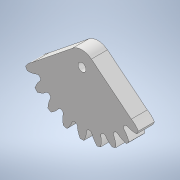
# Autodesk Inventor part: Pinion222
Saved by Autodesk Inventor 2022 (Build 260153000, 153)
## iProperties
Created: 2022-06-04
Part Number: Pinion222
Material: Generic
Document SubType Name: Modeling
Designer: frede
Density: 1 g/cm^3
Appearance: Default
Author: frede
Autodesk Inventor part; units mm, degrees
(part 1 of 2)
ref_plane "YZ Plane" through (0, 0, 0) normal (1, 0, 0) x (0, 1, 0)
ref_plane "XZ Plane" through (0, 0, 0) normal (0, 1, 0) x (-1, 0, 0)
ref_plane "XY Plane" through (0, 0, 0) normal (0, 0, 1) x (1, 0, 0)
sketch "Sketch1" plane through (0, 0, 0) normal (0, 0, 1) x (1, 0, 0)
  spline S0 degree 3 poles (-3.3489, 31.0344) (-3.2669, 30.9208) (-3.1027, 30.6937) (-2.8692, 30.344) (-2.6455, 29.988) (-2.4333, 29.625) (-2.2335, 29.255) (-2.0474, 28.8779) (-1.8767, 28.4936) (-1.7233, 28.102) (-1.5918, 27.7027) (-1.4824, 27.296) (-1.4363, 26.9482) (-1.3713, 26.6753) (-1.3031, 26.4761) (-1.2148, 26.2851) (-1.1055, 26.1048) (-0.9893, 25.973) (-0.8874, 25.8765) (-0.8022, 25.8147) (-0.714, 25.7572) (-0.6186, 25.7128) (-0.5212, 25.6728) (-0.4188, 25.6481) (-0.3154, 25.6283) (-0.1751, 25.6229) (0, 25.6264) (0.1751, 25.6229) (0.3154, 25.6283) (0.4188, 25.6481) (0.5212, 25.6728) (0.6186, 25.7128) (0.714, 25.7572) (0.8022, 25.8147) (0.8874, 25.8765) (0.9893, 25.973) (1.1055, 26.1048) (1.2148, 26.2851) (1.3031, 26.4761) (1.3713, 26.6753) (1.4363, 26.9482) (1.4824, 27.296) (1.5918, 27.7027) (1.7233, 28.102) (1.8767, 28.4936) (2.0474, 28.8779) (2.2335, 29.255) (2.4333, 29.625) (2.6455, 29.988) (2.8692, 30.344) (3.1027, 30.6937) (3.2669, 30.9208) (3.3489, 31.0344) knots 0 0 0 0 0.042039 0.084079 0.126119 0.168158 0.210197 0.252236 0.294274 0.336311 0.378346 0.420376 0.46241 0.483428 0.504444 0.525453 0.546459 0.567453 0.577965 0.588475 0.598984 0.609494 0.620001 0.63051 0.641019 0.651526 0.672547 0.693567 0.704074 0.714583 0.725092 0.735599 0.746109 0.756618 0.767128 0.77764 0.798635 0.81964 0.840649 0.861665 0.882683 0.924717 0.966747 1.008782 1.050819 1.092857 1.134896 1.176935 1.218975 1.261014 1.303054 1.345093 1.345093 1.345093 1.345093
  circle A0 centre (0, 0) radius 25.625 construction
  circle A1 centre (0, 0) radius 27.0162 construction
  circle A2 centre (0, 0) radius 28.75 construction
  circle A3 centre (0, 0) radius 31.2146
  point P0 (-3.1048, 30.6922)
  point P1 (-2.8708, 30.3429)
  point P2 (-2.6474, 29.9868)
  point P3 (-2.4354, 29.6238)
  point P4 (-2.2358, 29.2538)
  point P5 (-2.05, 28.8767)
  point P6 (-1.8796, 28.4924)
  point P7 (-1.7269, 28.1007)
  point P8 (-1.5955, 27.7015)
  point P9 (-1.4914, 27.2943)
  point P10 (-1.4177, 26.8804)
  point P11 (-1.368, 26.6762)
  point P12 (-1.2997, 26.4774)
  point P13 (-1.2113, 26.2869)
  point P14 (-1.1005, 26.1085)
  point P15 (-0.9631, 25.9497)
  point P16 (-0.8859, 25.8783)
  point P17 (-0.8017, 25.8154)
  point P18 (-0.7128, 25.7594)
  point P19 (-0.6182, 25.7135)
  point P20 (-0.5203, 25.6754)
  point P21 (-0.4186, 25.6489)
  point P22 (-0.3151, 25.6309)
  point P23 (-0.2102, 25.6249)
  point P24 (0, 25.625)
  point P25 (0.2102, 25.6249)
  point P26 (0.3151, 25.6309)
  point P27 (0.4186, 25.6489)
  point P28 (0.5203, 25.6754)
  point P29 (0.6182, 25.7135)
  point P30 (0.7128, 25.7594)
  point P31 (0.8017, 25.8154)
  point P32 (0.8859, 25.8783)
  point P33 (0.9631, 25.9497)
  point P34 (1.1005, 26.1085)
  point P35 (1.2113, 26.2869)
  point P36 (1.2997, 26.4774)
  point P37 (1.368, 26.6762)
  point P38 (1.4177, 26.8804)
  point P39 (1.4914, 27.2943)
  point P40 (1.5955, 27.7015)
  point P41 (1.7269, 28.1007)
  point P42 (1.8796, 28.4924)
  point P43 (2.05, 28.8767)
  point P44 (2.2358, 29.2538)
  point P45 (2.4354, 29.6238)
  point P46 (2.6474, 29.9868)
  point P47 (2.8708, 30.3429)
  point P48 (3.1048, 30.6922)
  constraints: 4 centre point, 2 point on circle, 107 other
extrude "Extrusion1" add sketch "Sketch1" against normal blind 8
extrude "Extrusion2" cut sketch "Sketch1" against normal through all contours A3 S0 picked at (-0.4102, 29.7407)
pattern_circular "Circular Pattern1" count 23 over 360 about axis through (0, 0, 0) along (0, 0, -1) of "Extrusion2"
sketch "Sketch3" plane through (0, 0, 0) normal (0, 0, 1) x (1, 0, 0)
  circle A0 centre (0, 0) radius 2
  dimension "d16" = 4
  constraints: 1 centre point, 1 coincident
  measures "d16" diameter of A0
extrude "Extrusion4" cut sketch "Sketch3" against normal through all
sketch "Sketch4" plane through (0, 0, -8) normal (0, 0, -1) x (-1, 0, 0)
  circle A0 centre (0, 0) radius 2 projected
  arc A1 (7.5436, -30.2893) -> (9.2925, -29.7993) centre (0, 0) ccw projected
  line L0 (0, 0) -> (0.9081, -31.2014) construction
  line L1 (0, 0) -> (26.1697, 16.142) construction
  circle A2 centre (0, 0) radius 7.5 construction
  circle A3 centre (0, 0) radius 2 projected
  spline S0 degree 5 poles (11.5977, 28.98) (11.5528, 28.9443) (11.5079, 28.9087) (11.4631, 28.8729) (11.3736, 28.8011) (11.2848, 28.7285) (11.2406, 28.692) (11.1527, 28.6184) (11.0656, 28.5437) (11.0223, 28.5061) (10.936, 28.4305) (10.8504, 28.3541) (10.8079, 28.3157) (10.7231, 28.2384) (10.6391, 28.1603) (10.5973, 28.121) (10.5142, 28.0419) (10.432, 27.962) (10.3911, 27.9218) (10.3097, 27.8409) (10.2294, 27.759) (10.1894, 27.7179) (10.1101, 27.6351) (10.0317, 27.5513) (9.9928, 27.5092) (9.9155, 27.4244) (9.8393, 27.3386) (9.8015, 27.2955) (9.7265, 27.2087) (9.6527, 27.1209) (9.6161, 27.0768) (9.5435, 26.9879) (9.4724, 26.898) (9.4371, 26.8527) (9.3674, 26.7616) (9.2993, 26.6693) (9.2655, 26.623) (9.1992, 26.5294) (9.1345, 26.4347) (9.1026, 26.387) (9.0395, 26.2912) (8.9784, 26.1941) (8.9484, 26.1452) (8.8896, 26.0467) (8.8341, 25.9463) (8.8071, 25.8957) (8.7566, 25.7927) (8.7081, 25.6886) (8.684, 25.6366) (8.6345, 25.533) (8.5814, 25.4313) (8.5535, 25.3811) (8.4945, 25.2826) (8.4291, 25.1882) (8.3946, 25.1423) (8.3227, 25.0526) (8.2443, 24.9687) (8.2037, 24.9279) (8.1183, 24.8511) (8.0248, 24.7838) (7.9755, 24.7547) (7.8775, 24.6942) (7.7704, 24.6518) (7.7164, 24.6331) (7.606, 24.5997) (7.4918, 24.5879) (7.4348, 24.5781) (7.32, 24.5847) (7.2058, 24.5928) (7.1497, 24.6085) (7.0395, 24.6378) (6.9295, 24.6711) (6.8743, 24.6853) (6.7637, 24.716) (6.6539, 24.7472) (6.5994, 24.7666) (6.4983, 24.8195) (6.3987, 24.8764) (6.3567, 24.9157) (6.2653, 24.9849) (6.1928, 25.0743) (6.1549, 25.1166) (6.0903, 25.2116) (6.0377, 25.3129) (6.0124, 25.3644) (5.9686, 25.4703) (5.9381, 25.5807) (5.9249, 25.6363) (5.9027, 25.7487) (5.8891, 25.8623) (5.8842, 25.9193) (5.8782, 26.0336) (5.8798, 26.1481) (5.8824, 26.2052) (5.8906, 26.3193) (5.9025, 26.4331) (5.909, 26.4899) (5.9215, 26.6036) (5.931, 26.7175) (5.934, 26.7746) (5.9383, 26.8889) (5.939, 27.0032) (5.9386, 27.0604) (5.9366, 27.1747) (5.9323, 27.2889) (5.9297, 27.346) (5.9234, 27.4601) (5.9152, 27.5741) (5.9104, 27.631) (5.9, 27.7448) (5.8876, 27.8584) (5.881, 27.9151) (5.8669, 28.0285) (5.851, 28.1417) (5.8426, 28.1982) (5.8251, 28.3111) (5.8061, 28.4238) (5.7962, 28.4801) (5.7756, 28.5925) (5.7537, 28.7046) (5.7423, 28.7606) (5.7189, 28.8725) (5.6941, 28.984) (5.6814, 29.0397) (5.6553, 29.1509) (5.6279, 29.2619) (5.6139, 29.3173) (5.5852, 29.4279) (5.5553, 29.5382) (5.5401, 29.5932) (5.509, 29.7032) (5.4768, 29.8128) (5.4604, 29.8676) (5.4271, 29.9769) (5.3928, 30.0859) (5.3754, 30.1403) (5.3399, 30.2489) (5.3031, 30.3571) (5.2844, 30.4111) (5.2464, 30.5188) (5.2074, 30.6262) (5.1877, 30.6799) (5.168, 30.7335) (5.1482, 30.7871) knots 0 0 0 0 0 0 0.021315 0.021315 0.021315 0.04263 0.04263 0.04263 0.063945 0.063945 0.063945 0.08526 0.08526 0.08526 0.106575 0.106575 0.106575 0.12789 0.12789 0.12789 0.149204 0.149204 0.149204 0.170519 0.170519 0.170519 0.191835 0.191835 0.191835 0.21315 0.21315 0.21315 0.234465 0.234465 0.234465 0.255779 0.255779 0.255779 0.277094 0.277094 0.277094 0.298412 0.298412 0.298412 0.319724 0.319724 0.319724 0.341052 0.341052 0.341052 0.362374 0.362374 0.362374 0.383705 0.383705 0.383705 0.405045 0.405045 0.405045 0.42637 0.42637 0.42637 0.447676 0.447676 0.447676 0.468973 0.468973 0.468973 0.490261 0.490261 0.490261 0.511544 0.511544 0.511544 0.532795 0.532795 0.532795 0.554 0.554 0.554 0.575212 0.575212 0.575212 0.596458 0.596458 0.596458 0.617711 0.617711 0.617711 0.63897 0.63897 0.63897 0.660221 0.660221 0.660221 0.681474 0.681474 0.681474 0.702716 0.702716 0.702716 0.723962 0.723962 0.723962 0.745198 0.745198 0.745198 0.76643 0.76643 0.76643 0.787663 0.787663 0.787663 0.808897 0.808897 0.808897 0.830131 0.830131 0.830131 0.851365 0.851365 0.851365 0.872598 0.872598 0.872598 0.893831 0.893831 0.893831 0.915065 0.915065 0.915065 0.936299 0.936299 0.936299 0.957533 0.957533 0.957533 0.978766 0.978766 0.978766 1 1 1 1 1 1 projected
  arc A4 (5.1482, 30.7871) -> (3.3489, 31.0344) centre (0, 0) ccw projected
  spline S1 degree 5 poles (3.3489, 31.0344) (3.3153, 30.9879) (3.2817, 30.9415) (3.2482, 30.8949) (3.1814, 30.8017) (3.1155, 30.7078) (3.0828, 30.6607) (3.018, 30.5661) (2.9543, 30.4707) (2.9227, 30.4228) (2.86, 30.3267) (2.7982, 30.2301) (2.7676, 30.1816) (2.7068, 30.0843) (2.647, 29.9864) (2.6174, 29.9373) (2.5587, 29.8388) (2.5011, 29.7396) (2.4725, 29.6898) (2.416, 29.59) (2.3607, 29.4895) (2.3334, 29.4391) (2.2793, 29.3379) (2.2265, 29.2361) (2.2004, 29.1851) (2.1488, 29.0826) (2.0986, 28.9795) (2.0738, 28.9277) (2.025, 28.8239) (1.9776, 28.7195) (1.9543, 28.6671) (1.9084, 28.5619) (1.8641, 28.4561) (1.8424, 28.403) (1.7998, 28.2965) (1.7591, 28.1893) (1.7392, 28.1355) (1.7005, 28.0275) (1.6638, 27.9189) (1.6459, 27.8644) (1.611, 27.7551) (1.5784, 27.6451) (1.5627, 27.5899) (1.5327, 27.4792) (1.5063, 27.3676) (1.494, 27.3115) (1.4731, 27.1987) (1.4545, 27.0855) (1.4453, 27.0288) (1.4256, 26.9158) (1.4019, 26.8035) (1.3885, 26.7476) (1.3583, 26.6369) (1.3208, 26.5283) (1.2999, 26.4748) (1.2549, 26.369) (1.2021, 26.2671) (1.174, 26.2168) (1.1125, 26.1199) (1.0407, 26.0298) (1.001, 25.9885) (0.923, 25.9038) (0.8313, 25.8341) (0.7843, 25.8015) (0.6871, 25.7395) (0.5802, 25.6974) (0.528, 25.6726) (0.4156, 25.648) (0.3035, 25.625) (0.2453, 25.6249) (0.1313, 25.6234) (0.0163, 25.6258) (-0.0407, 25.6246) (-0.1554, 25.6243) (-0.2695, 25.6247) (-0.3273, 25.6287) (-0.4389, 25.6524) (-0.5501, 25.6803) (-0.6012, 25.7068) (-0.7079, 25.7487) (-0.8018, 25.8153) (-0.8498, 25.8458) (-0.9376, 25.9198) (-1.0156, 26.0032) (-1.0538, 26.046) (-1.1245, 26.1361) (-1.1837, 26.2342) (-1.2114, 26.2842) (-1.2631, 26.3864) (-1.3068, 26.4921) (-1.3269, 26.5457) (-1.3636, 26.6542) (-1.3929, 26.7648) (-1.4058, 26.8205) (-1.4288, 26.9326) (-1.4479, 27.0453) (-1.4571, 27.1018) (-1.4757, 27.2146) (-1.4972, 27.3269) (-1.5097, 27.3827) (-1.5364, 27.4939) (-1.5667, 27.6042) (-1.5824, 27.6591) (-1.6152, 27.7686) (-1.6502, 27.8775) (-1.6681, 27.9317) (-1.7049, 28.0399) (-1.7435, 28.1474) (-1.7635, 28.201) (-1.8042, 28.3077) (-1.8468, 28.4138) (-1.8685, 28.4666) (-1.9127, 28.572) (-1.9585, 28.6767) (-1.9818, 28.7289) (-2.0291, 28.8329) (-2.0779, 28.9362) (-2.1026, 28.9877) (-2.1527, 29.0904) (-2.2041, 29.1925) (-2.2302, 29.2433) (-2.2829, 29.3447) (-2.3368, 29.4455) (-2.3641, 29.4956) (-2.4193, 29.5957) (-2.4756, 29.6951) (-2.504, 29.7447) (-2.5615, 29.8435) (-2.62, 29.9416) (-2.6495, 29.9905) (-2.7091, 30.088) (-2.7697, 30.1849) (-2.8002, 30.2332) (-2.8618, 30.3295) (-2.9243, 30.4252) (-2.9557, 30.4729) (-3.0192, 30.5679) (-3.0838, 30.6621) (-3.1164, 30.7091) (-3.1821, 30.8026) (-3.2486, 30.8955) (-3.282, 30.9418) (-3.3155, 30.9881) (-3.3489, 31.0344) knots 0 0 0 0 0 0 0.021315 0.021315 0.021315 0.04263 0.04263 0.04263 0.063945 0.063945 0.063945 0.08526 0.08526 0.08526 0.106575 0.106575 0.106575 0.12789 0.12789 0.12789 0.149204 0.149204 0.149204 0.170519 0.170519 0.170519 0.191835 0.191835 0.191835 0.21315 0.21315 0.21315 0.234465 0.234465 0.234465 0.255779 0.255779 0.255779 0.277094 0.277094 0.277094 0.298412 0.298412 0.298412 0.319724 0.319724 0.319724 0.341052 0.341052 0.341052 0.362374 0.362374 0.362374 0.383705 0.383705 0.383705 0.405045 0.405045 0.405045 0.42637 0.42637 0.42637 0.447676 0.447676 0.447676 0.468973 0.468973 0.468973 0.490261 0.490261 0.490261 0.511544 0.511544 0.511544 0.532795 0.532795 0.532795 0.554 0.554 0.554 0.575212 0.575212 0.575212 0.596458 0.596458 0.596458 0.617711 0.617711 0.617711 0.63897 0.63897 0.63897 0.660221 0.660221 0.660221 0.681474 0.681474 0.681474 0.702716 0.702716 0.702716 0.723962 0.723962 0.723962 0.745198 0.745198 0.745198 0.76643 0.76643 0.76643 0.787663 0.787663 0.787663 0.808897 0.808897 0.808897 0.830131 0.830131 0.830131 0.851365 0.851365 0.851365 0.872598 0.872598 0.872598 0.893831 0.893831 0.893831 0.915065 0.915065 0.915065 0.936299 0.936299 0.936299 0.957533 0.957533 0.957533 0.978766 0.978766 0.978766 1 1 1 1 1 1 projected
  arc A5 (-3.3489, 31.0344) -> (-5.1482, 30.7871) centre (0, 0) ccw projected
  spline S2 degree 5 poles (-5.1482, 30.7871) (-5.168, 30.7333) (-5.1879, 30.6795) (-5.2076, 30.6256) (-5.2468, 30.5178) (-5.2849, 30.4096) (-5.3037, 30.3554) (-5.3406, 30.2468) (-5.3762, 30.1378) (-5.3936, 30.0832) (-5.4281, 29.9737) (-5.4615, 29.864) (-5.4779, 29.8091) (-5.5102, 29.699) (-5.5414, 29.5886) (-5.5567, 29.5333) (-5.5866, 29.4226) (-5.6153, 29.3115) (-5.6294, 29.2559) (-5.6568, 29.1446) (-5.683, 29.0329) (-5.6957, 28.977) (-5.7205, 28.865) (-5.7439, 28.7527) (-5.7553, 28.6965) (-5.7773, 28.5839) (-5.7978, 28.471) (-5.8077, 28.4145) (-5.8267, 28.3014) (-5.8442, 28.188) (-5.8525, 28.1313) (-5.8683, 28.0177) (-5.8824, 27.9038) (-5.889, 27.8468) (-5.9012, 27.7328) (-5.9115, 27.6186) (-5.9162, 27.5614) (-5.9243, 27.447) (-5.9304, 27.3324) (-5.9329, 27.2751) (-5.9369, 27.1605) (-5.9387, 27.0458) (-5.9389, 26.9884) (-5.938, 26.8737) (-5.9332, 26.7591) (-5.93, 26.7018) (-5.9197, 26.5875) (-5.907, 26.4735) (-5.9006, 26.4165) (-5.889, 26.3023) (-5.8816, 26.1877) (-5.8794, 26.1304) (-5.8786, 26.0156) (-5.8854, 25.9009) (-5.8911, 25.8438) (-5.9059, 25.7298) (-5.9293, 25.6174) (-5.9428, 25.5614) (-5.9758, 25.4514) (-6.0207, 25.3453) (-6.0477, 25.2948) (-6.1, 25.1922) (-6.1695, 25.1004) (-6.2059, 25.0563) (-6.2829, 24.9704) (-6.3743, 24.901) (-6.418, 24.863) (-6.5195, 24.809) (-6.6213, 24.7566) (-6.6773, 24.7409) (-6.7867, 24.7086) (-6.898, 24.6799) (-6.9526, 24.6634) (-7.063, 24.6321) (-7.173, 24.6018) (-7.2297, 24.59) (-7.3435, 24.5827) (-7.4582, 24.5796) (-7.5146, 24.5913) (-7.6285, 24.6029) (-7.7369, 24.6416) (-7.7914, 24.6581) (-7.8959, 24.7057) (-7.9935, 24.7649) (-8.0418, 24.7958) (-8.1342, 24.8635) (-8.2177, 24.942) (-8.2579, 24.9827) (-8.3352, 25.0671) (-8.4059, 25.1571) (-8.4397, 25.2033) (-8.5042, 25.2979) (-8.5623, 25.3965) (-8.5898, 25.4467) (-8.6421, 25.5484) (-8.691, 25.6518) (-8.715, 25.7037) (-8.7634, 25.8073) (-8.8144, 25.9096) (-8.8415, 25.96) (-8.8972, 26.0598) (-8.9561, 26.1579) (-8.9861, 26.2065) (-9.0472, 26.3031) (-9.1102, 26.3985) (-9.1421, 26.4459) (-9.2067, 26.5401) (-9.273, 26.6333) (-9.3066, 26.6794) (-9.3747, 26.7712) (-9.4443, 26.8619) (-9.4794, 26.9069) (-9.5504, 26.9964) (-9.6228, 27.0849) (-9.6593, 27.1288) (-9.7329, 27.2162) (-9.8077, 27.3026) (-9.8454, 27.3455) (-9.9214, 27.4309) (-9.9984, 27.5153) (-10.0372, 27.5572) (-10.1153, 27.6406) (-10.1944, 27.7231) (-10.2343, 27.764) (-10.3144, 27.8455) (-10.3954, 27.9261) (-10.4362, 27.9661) (-10.5182, 28.0457) (-10.601, 28.1244) (-10.6426, 28.1636) (-10.7263, 28.2414) (-10.8108, 28.3183) (-10.8532, 28.3566) (-10.9385, 28.4327) (-11.0244, 28.5079) (-11.0676, 28.5454) (-11.1543, 28.6198) (-11.242, 28.6931) (-11.286, 28.7295) (-11.3745, 28.8018) (-11.4636, 28.8733) (-11.5083, 28.9089) (-11.553, 28.9445) (-11.5977, 28.98) knots 0 0 0 0 0 0 0.021315 0.021315 0.021315 0.04263 0.04263 0.04263 0.063945 0.063945 0.063945 0.08526 0.08526 0.08526 0.106575 0.106575 0.106575 0.12789 0.12789 0.12789 0.149204 0.149204 0.149204 0.170519 0.170519 0.170519 0.191835 0.191835 0.191835 0.21315 0.21315 0.21315 0.234465 0.234465 0.234465 0.255779 0.255779 0.255779 0.277094 0.277094 0.277094 0.298412 0.298412 0.298412 0.319724 0.319724 0.319724 0.341052 0.341052 0.341052 0.362374 0.362374 0.362374 0.383705 0.383705 0.383705 0.405045 0.405045 0.405045 0.42637 0.42637 0.42637 0.447676 0.447676 0.447676 0.468973 0.468973 0.468973 0.490261 0.490261 0.490261 0.511544 0.511544 0.511544 0.532795 0.532795 0.532795 0.554 0.554 0.554 0.575212 0.575212 0.575212 0.596458 0.596458 0.596458 0.617711 0.617711 0.617711 0.63897 0.63897 0.63897 0.660221 0.660221 0.660221 0.681474 0.681474 0.681474 0.702716 0.702716 0.702716 0.723962 0.723962 0.723962 0.745198 0.745198 0.745198 0.76643 0.76643 0.76643 0.787663 0.787663 0.787663 0.808897 0.808897 0.808897 0.830131 0.830131 0.830131 0.851365 0.851365 0.851365 0.872598 0.872598 0.872598 0.893831 0.893831 0.893831 0.915065 0.915065 0.915065 0.936299 0.936299 0.936299 0.957533 0.957533 0.957533 0.978766 0.978766 0.978766 1 1 1 1 1 1 projected
  arc A6 (-11.5977, 28.98) -> (-13.2636, 28.2565) centre (0, 0) ccw projected
  spline S3 degree 5 poles (-13.2636, 28.2565) (-13.2681, 28.1993) (-13.2727, 28.1421) (-13.2772, 28.0849) (-13.2858, 27.9706) (-13.2933, 27.8561) (-13.2968, 27.7989) (-13.303, 27.6843) (-13.3079, 27.5697) (-13.31, 27.5124) (-13.3136, 27.3978) (-13.3162, 27.2831) (-13.3172, 27.2257) (-13.3186, 27.111) (-13.3188, 26.9963) (-13.3186, 26.939) (-13.3176, 26.8243) (-13.3153, 26.7096) (-13.3138, 26.6523) (-13.3102, 26.5376) (-13.3052, 26.423) (-13.3024, 26.3657) (-13.296, 26.2512) (-13.2883, 26.1368) (-13.2841, 26.0796) (-13.2749, 25.9652) (-13.2642, 25.851) (-13.2585, 25.7939) (-13.2463, 25.6799) (-13.2325, 25.566) (-13.2252, 25.5091) (-13.2098, 25.3954) (-13.1926, 25.282) (-13.1836, 25.2254) (-13.1646, 25.1123) (-13.1437, 24.9995) (-13.1328, 24.9432) (-13.1097, 24.8308) (-13.0846, 24.7189) (-13.0716, 24.663) (-13.0446, 24.5515) (-13.0153, 24.4406) (-13.0001, 24.3853) (-12.9682, 24.2751) (-12.9327, 24.166) (-12.9141, 24.1117) (-12.8734, 24.0045) (-12.8304, 23.8981) (-12.8089, 23.8449) (-12.7669, 23.7381) (-12.7289, 23.6298) (-12.7112, 23.5751) (-12.6795, 23.4648) (-12.6551, 23.3526) (-12.6452, 23.296) (-12.6287, 23.1822) (-12.6209, 23.0677) (-12.6188, 23.0101) (-12.6209, 22.8953) (-12.6355, 22.7811) (-12.6479, 22.7251) (-12.6706, 22.6123) (-12.7127, 22.5051) (-12.7359, 22.4528) (-12.7868, 22.3493) (-12.8562, 22.2578) (-12.8879, 22.2095) (-12.9711, 22.1301) (-13.055, 22.0522) (-13.1047, 22.0219) (-13.2014, 21.9613) (-13.3008, 21.9036) (-13.3489, 21.873) (-13.4467, 21.8132) (-13.5445, 21.7542) (-13.5959, 21.7276) (-13.7035, 21.6899) (-13.8131, 21.6559) (-13.8706, 21.652) (-13.9834, 21.6324) (-14.0982, 21.6405) (-14.1551, 21.6416) (-14.2686, 21.6592) (-14.3786, 21.69) (-14.4334, 21.7066) (-14.5407, 21.7469) (-14.6422, 21.7999) (-14.6919, 21.8283) (-14.7891, 21.8887) (-14.8815, 21.9564) (-14.9265, 21.9917) (-15.0141, 22.0653) (-15.0967, 22.1446) (-15.1367, 22.1855) (-15.2145, 22.2694) (-15.2895, 22.3557) (-15.3266, 22.3992) (-15.4011, 22.486) (-15.4779, 22.5707) (-15.5176, 22.6119) (-15.5981, 22.693) (-15.6813, 22.7715) (-15.7233, 22.8103) (-15.8082, 22.8868) (-15.8946, 22.9617) (-15.9381, 22.9987) (-16.0258, 23.072) (-16.1147, 23.1438) (-16.1595, 23.1792) (-16.2498, 23.2492) (-16.3413, 23.3177) (-16.3873, 23.3516) (-16.4798, 23.4187) (-16.5733, 23.4843) (-16.6203, 23.5168) (-16.7148, 23.5811) (-16.8102, 23.6441) (-16.8581, 23.6752) (-16.9542, 23.7369) (-17.0512, 23.7974) (-17.0999, 23.8273) (-17.1976, 23.8866) (-17.296, 23.9446) (-17.3454, 23.9733) (-17.4445, 24.0302) (-17.5443, 24.0858) (-17.5943, 24.1134) (-17.6948, 24.1679) (-17.7958, 24.2214) (-17.8464, 24.2478) (-17.948, 24.3002) (-18.0501, 24.3515) (-18.1013, 24.3769) (-18.2039, 24.4271) (-18.307, 24.4764) (-18.3586, 24.5009) (-18.4622, 24.5491) (-18.5664, 24.596) (-18.6186, 24.6192) (-18.7233, 24.665) (-18.8284, 24.7098) (-18.8811, 24.732) (-18.9337, 24.7542) (-18.9864, 24.7764) knots 0 0 0 0 0 0 0.021315 0.021315 0.021315 0.04263 0.04263 0.04263 0.063945 0.063945 0.063945 0.08526 0.08526 0.08526 0.106575 0.106575 0.106575 0.12789 0.12789 0.12789 0.149204 0.149204 0.149204 0.170519 0.170519 0.170519 0.191835 0.191835 0.191835 0.21315 0.21315 0.21315 0.234465 0.234465 0.234465 0.255779 0.255779 0.255779 0.277094 0.277094 0.277094 0.298412 0.298412 0.298412 0.319724 0.319724 0.319724 0.341052 0.341052 0.341052 0.362374 0.362374 0.362374 0.383705 0.383705 0.383705 0.405045 0.405045 0.405045 0.42637 0.42637 0.42637 0.447676 0.447676 0.447676 0.468973 0.468973 0.468973 0.490261 0.490261 0.490261 0.511544 0.511544 0.511544 0.532795 0.532795 0.532795 0.554 0.554 0.554 0.575212 0.575212 0.575212 0.596458 0.596458 0.596458 0.617711 0.617711 0.617711 0.63897 0.63897 0.63897 0.660221 0.660221 0.660221 0.681474 0.681474 0.681474 0.702716 0.702716 0.702716 0.723962 0.723962 0.723962 0.745198 0.745198 0.745198 0.76643 0.76643 0.76643 0.787663 0.787663 0.787663 0.808897 0.808897 0.808897 0.830131 0.830131 0.830131 0.851365 0.851365 0.851365 0.872598 0.872598 0.872598 0.893831 0.893831 0.893831 0.915065 0.915065 0.915065 0.936299 0.936299 0.936299 0.957533 0.957533 0.957533 0.978766 0.978766 0.978766 1 1 1 1 1 1 projected
  arc A7 (-18.9864, 24.7764) -> (-20.3952, 23.6302) centre (0, 0) ccw projected
  spline S4 degree 5 poles (-20.3952, 23.6302) (-20.3842, 23.5739) (-20.3732, 23.5176) (-20.3621, 23.4613) (-20.3395, 23.3489) (-20.3159, 23.2366) (-20.3038, 23.1806) (-20.2789, 23.0686) (-20.2526, 22.9569) (-20.2392, 22.9012) (-20.2117, 22.7898) (-20.1833, 22.6787) (-20.1688, 22.6232) (-20.1392, 22.5124) (-20.1084, 22.4019) (-20.0927, 22.3467) (-20.0608, 22.2365) (-20.0277, 22.1267) (-20.0108, 22.0719) (-19.9764, 21.9625) (-19.9407, 21.8535) (-19.9225, 21.7991) (-19.8855, 21.6905) (-19.8471, 21.5824) (-19.8276, 21.5285) (-19.7879, 21.4208) (-19.7468, 21.3138) (-19.7259, 21.2603) (-19.6834, 21.1538) (-19.6394, 21.0479) (-19.6171, 20.995) (-19.5715, 20.8898) (-19.5244, 20.7852) (-19.5004, 20.7331) (-19.4516, 20.6293) (-19.4011, 20.5263) (-19.3754, 20.475) (-19.3229, 20.373) (-19.2685, 20.272) (-19.2409, 20.2218) (-19.1848, 20.1217) (-19.1267, 20.0228) (-19.0971, 19.9736) (-19.0367, 19.8761) (-18.9731, 19.7807) (-18.9405, 19.7334) (-18.8723, 19.6411) (-18.8023, 19.5503) (-18.7672, 19.5049) (-18.6979, 19.4133) (-18.6321, 19.3193) (-18.6004, 19.2715) (-18.54, 19.1738) (-18.4863, 19.0723) (-18.4615, 19.0205) (-18.4149, 18.9154) (-18.3765, 18.8072) (-18.3589, 18.7524) (-18.33, 18.6412) (-18.3132, 18.5273) (-18.3101, 18.4701) (-18.3014, 18.3553) (-18.3131, 18.2407) (-18.3213, 18.1841) (-18.3424, 18.0707) (-18.3845, 17.9639) (-18.4021, 17.9087) (-18.4608, 17.8099) (-18.5205, 17.7122) (-18.5602, 17.6697) (-18.6369, 17.5853) (-18.7171, 17.5029) (-18.7551, 17.4604) (-18.8332, 17.3764) (-18.9114, 17.2932) (-18.9538, 17.2538) (-19.0472, 17.1884) (-19.1436, 17.1261) (-19.1978, 17.1068) (-19.3012, 17.0575) (-19.414, 17.0343) (-19.4691, 17.0201) (-19.5831, 17.0064) (-19.6973, 17.0063) (-19.7546, 17.0076) (-19.8687, 17.0174) (-19.9808, 17.0411) (-20.0363, 17.055) (-20.1462, 17.087) (-20.2534, 17.1272) (-20.3063, 17.1491) (-20.4105, 17.1963) (-20.5114, 17.2504) (-20.5609, 17.279) (-20.6585, 17.3387) (-20.754, 17.4017) (-20.8015, 17.4335) (-20.8966, 17.497) (-20.9934, 17.5579) (-21.0428, 17.5868) (-21.1422, 17.6432) (-21.2434, 17.6963) (-21.2944, 17.7223) (-21.3968, 17.7731) (-21.5002, 17.8219) (-21.5521, 17.8458) (-21.6562, 17.8927) (-21.7612, 17.9379) (-21.814, 17.9598) (-21.9198, 18.0029) (-22.0263, 18.0442) (-22.0798, 18.0644) (-22.187, 18.104) (-22.2947, 18.142) (-22.3488, 18.1606) (-22.4571, 18.197) (-22.5659, 18.2319) (-22.6204, 18.249) (-22.7297, 18.2825) (-22.8393, 18.3146) (-22.8943, 18.3303) (-23.0044, 18.3609) (-23.1148, 18.3903) (-23.1701, 18.4046) (-23.2809, 18.4326) (-23.392, 18.4593) (-23.4476, 18.4723) (-23.559, 18.4977) (-23.6707, 18.522) (-23.7266, 18.5338) (-23.8385, 18.5568) (-23.9507, 18.5786) (-24.0068, 18.5893) (-24.1192, 18.61) (-24.2318, 18.6296) (-24.2881, 18.6392) (-24.4009, 18.6577) (-24.5138, 18.6748) (-24.5704, 18.683) (-24.6835, 18.6988) (-24.7968, 18.7136) (-24.8535, 18.7208) (-24.9102, 18.728) (-24.9669, 18.7351) knots 0 0 0 0 0 0 0.021315 0.021315 0.021315 0.04263 0.04263 0.04263 0.063945 0.063945 0.063945 0.08526 0.08526 0.08526 0.106575 0.106575 0.106575 0.12789 0.12789 0.12789 0.149204 0.149204 0.149204 0.170519 0.170519 0.170519 0.191835 0.191835 0.191835 0.21315 0.21315 0.21315 0.234465 0.234465 0.234465 0.255779 0.255779 0.255779 0.277094 0.277094 0.277094 0.298412 0.298412 0.298412 0.319724 0.319724 0.319724 0.341052 0.341052 0.341052 0.362374 0.362374 0.362374 0.383705 0.383705 0.383705 0.405045 0.405045 0.405045 0.42637 0.42637 0.42637 0.447676 0.447676 0.447676 0.468973 0.468973 0.468973 0.490261 0.490261 0.490261 0.511544 0.511544 0.511544 0.532795 0.532795 0.532795 0.554 0.554 0.554 0.575212 0.575212 0.575212 0.596458 0.596458 0.596458 0.617711 0.617711 0.617711 0.63897 0.63897 0.63897 0.660221 0.660221 0.660221 0.681474 0.681474 0.681474 0.702716 0.702716 0.702716 0.723962 0.723962 0.723962 0.745198 0.745198 0.745198 0.76643 0.76643 0.76643 0.787663 0.787663 0.787663 0.808897 0.808897 0.808897 0.830131 0.830131 0.830131 0.851365 0.851365 0.851365 0.872598 0.872598 0.872598 0.893831 0.893831 0.893831 0.915065 0.915065 0.915065 0.936299 0.936299 0.936299 0.957533 0.957533 0.957533 0.978766 0.978766 0.978766 1 1 1 1 1 1 projected
  arc A8 (-24.9669, 18.7351) -> (-26.0143, 17.2513) centre (0, 0) ccw projected
  spline S5 degree 5 poles (-26.0143, 17.2513) (-25.9885, 17.2001) (-25.9627, 17.1489) (-25.9368, 17.0977) (-25.8847, 16.9955) (-25.8317, 16.8938) (-25.8049, 16.8431) (-25.7507, 16.742) (-25.6953, 16.6415) (-25.6673, 16.5915) (-25.6108, 16.4916) (-25.5535, 16.3923) (-25.5245, 16.3428) (-25.4661, 16.2441) (-25.4067, 16.146) (-25.3767, 16.0971) (-25.3162, 15.9996) (-25.2547, 15.9028) (-25.2236, 15.8546) (-25.161, 15.7585) (-25.0972, 15.6632) (-25.065, 15.6157) (-25.0001, 15.5211) (-24.934, 15.4274) (-24.9007, 15.3807) (-24.8334, 15.2878) (-24.765, 15.1957) (-24.7304, 15.15) (-24.6607, 15.0588) (-24.5898, 14.9687) (-24.554, 14.9239) (-24.4817, 14.8348) (-24.4082, 14.7468) (-24.371, 14.7031) (-24.296, 14.6163) (-24.2195, 14.5308) (-24.181, 14.4883) (-24.1029, 14.4043) (-24.0233, 14.3217) (-23.9832, 14.2808) (-23.9021, 14.1996) (-23.8195, 14.12) (-23.7778, 14.0806) (-23.6932, 14.003) (-23.6063, 13.9283) (-23.5622, 13.8916) (-23.4716, 13.8211) (-23.3796, 13.7525) (-23.3336, 13.7183) (-23.2422, 13.6488) (-23.1535, 13.576) (-23.11, 13.5385) (-23.0255, 13.4607) (-22.9464, 13.3775) (-22.9085, 13.3343) (-22.8353, 13.2457) (-22.7691, 13.1519) (-22.7374, 13.1038) (-22.6796, 13.0046) (-22.6327, 12.8994) (-22.6142, 12.8451) (-22.575, 12.737) (-22.5552, 12.6235) (-22.5479, 12.5667) (-22.5377, 12.4519) (-22.5494, 12.3377) (-22.5514, 12.2798) (-22.5812, 12.1688) (-22.6124, 12.0586) (-22.6391, 12.0069) (-22.6903, 11.905) (-22.7452, 11.804) (-22.7704, 11.7529) (-22.8229, 11.6509) (-22.8758, 11.5497) (-22.9059, 11.5003) (-22.9783, 11.4121) (-23.0542, 11.3261) (-23.1013, 11.293) (-23.1876, 11.2176) (-23.2898, 11.1648) (-23.3391, 11.1363) (-23.4452, 11.0923) (-23.5551, 11.0614) (-23.6106, 11.0472) (-23.7232, 11.0259) (-23.8375, 11.0184) (-23.8947, 11.0168) (-24.0092, 11.018) (-24.1232, 11.0278) (-24.18, 11.0346) (-24.2932, 11.052) (-24.4049, 11.0768) (-24.4603, 11.091) (-24.5704, 11.1222) (-24.6793, 11.157) (-24.7336, 11.1749) (-24.8424, 11.2103) (-24.952, 11.2428) (-25.0073, 11.2574) (-25.1183, 11.2848) (-25.2301, 11.3087) (-25.2861, 11.32) (-25.3985, 11.3412) (-25.5112, 11.3603) (-25.5676, 11.3694) (-25.6806, 11.3865) (-25.7938, 11.4016) (-25.8506, 11.4085) (-25.9641, 11.4214) (-26.0778, 11.4324) (-26.1347, 11.4375) (-26.2486, 11.4467) (-26.3627, 11.4542) (-26.4197, 11.4575) (-26.5338, 11.4634) (-26.648, 11.4677) (-26.7051, 11.4694) (-26.8194, 11.4722) (-26.9336, 11.4734) (-26.9907, 11.4737) (-27.105, 11.4736) (-27.2193, 11.472) (-27.2764, 11.4709) (-27.3906, 11.4679) (-27.5048, 11.4637) (-27.5619, 11.4612) (-27.676, 11.4556) (-27.7901, 11.4488) (-27.8471, 11.4451) (-27.9611, 11.4371) (-28.075, 11.4279) (-28.1319, 11.423) (-28.2457, 11.4126) (-28.3594, 11.4011) (-28.4162, 11.3952) (-28.5298, 11.3825) (-28.6432, 11.3685) (-28.6999, 11.3612) (-28.8131, 11.3459) (-28.9262, 11.3296) (-28.9827, 11.3212) (-29.0392, 11.3128) (-29.0957, 11.3044) knots 0 0 0 0 0 0 0.021315 0.021315 0.021315 0.04263 0.04263 0.04263 0.063945 0.063945 0.063945 0.08526 0.08526 0.08526 0.106575 0.106575 0.106575 0.12789 0.12789 0.12789 0.149204 0.149204 0.149204 0.170519 0.170519 0.170519 0.191835 0.191835 0.191835 0.21315 0.21315 0.21315 0.234465 0.234465 0.234465 0.255779 0.255779 0.255779 0.277094 0.277094 0.277094 0.298412 0.298412 0.298412 0.319724 0.319724 0.319724 0.341052 0.341052 0.341052 0.362374 0.362374 0.362374 0.383705 0.383705 0.383705 0.405045 0.405045 0.405045 0.42637 0.42637 0.42637 0.447676 0.447676 0.447676 0.468973 0.468973 0.468973 0.490261 0.490261 0.490261 0.511544 0.511544 0.511544 0.532795 0.532795 0.532795 0.554 0.554 0.554 0.575212 0.575212 0.575212 0.596458 0.596458 0.596458 0.617711 0.617711 0.617711 0.63897 0.63897 0.63897 0.660221 0.660221 0.660221 0.681474 0.681474 0.681474 0.702716 0.702716 0.702716 0.723962 0.723962 0.723962 0.745198 0.745198 0.745198 0.76643 0.76643 0.76643 0.787663 0.787663 0.787663 0.808897 0.808897 0.808897 0.830131 0.830131 0.830131 0.851365 0.851365 0.851365 0.872598 0.872598 0.872598 0.893831 0.893831 0.893831 0.915065 0.915065 0.915065 0.936299 0.936299 0.936299 0.957533 0.957533 0.957533 0.978766 0.978766 0.978766 1 1 1 1 1 1 projected
  arc A9 (-29.0957, 11.3044) -> (-29.7039, 9.593) centre (0, 0) ccw projected
  spline S6 degree 5 poles (-29.7039, 9.593) (-29.6653, 9.5507) (-29.6266, 9.5083) (-29.5879, 9.466) (-29.5102, 9.3817) (-29.4317, 9.298) (-29.3922, 9.2564) (-29.3127, 9.1737) (-29.2323, 9.0919) (-29.1918, 9.0513) (-29.1105, 8.9704) (-29.0285, 8.8902) (-28.9872, 8.8503) (-28.9044, 8.771) (-28.8207, 8.6926) (-28.7786, 8.6536) (-28.6941, 8.576) (-28.6087, 8.4994) (-28.5658, 8.4614) (-28.4795, 8.3858) (-28.3924, 8.3112) (-28.3486, 8.2741) (-28.2606, 8.2006) (-28.1716, 8.1282) (-28.127, 8.0922) (-28.0371, 8.0209) (-27.9464, 7.9507) (-27.9008, 7.916) (-27.8091, 7.847) (-27.7164, 7.7794) (-27.6699, 7.7459) (-27.5763, 7.6796) (-27.4817, 7.6147) (-27.4341, 7.5826) (-27.3385, 7.5193) (-27.2418, 7.4576) (-27.1932, 7.4271) (-27.0953, 7.3673) (-26.9964, 7.3092) (-26.9467, 7.2806) (-26.8468, 7.2243) (-26.7457, 7.1699) (-26.6949, 7.1433) (-26.5926, 7.0914) (-26.4887, 7.0429) (-26.4363, 7.0194) (-26.3301, 6.976) (-26.223, 6.9348) (-26.1694, 6.9142) (-26.0627, 6.872) (-25.9576, 6.8259) (-25.9057, 6.8015) (-25.8034, 6.7494) (-25.7047, 6.6905) (-25.6566, 6.6592) (-25.5622, 6.5936) (-25.4731, 6.5211) (-25.4296, 6.4834) (-25.3472, 6.4035) (-25.2736, 6.3148) (-25.2412, 6.2676) (-25.1742, 6.174) (-25.1246, 6.07) (-25.1023, 6.0174) (-25.0614, 5.9095) (-25.0418, 5.7964) (-25.0282, 5.7402) (-25.0269, 5.6252) (-25.0273, 5.5107) (-25.0391, 5.4537) (-25.0608, 5.3418) (-25.0864, 5.2297) (-25.0969, 5.1737) (-25.1199, 5.0613) (-25.1436, 4.9496) (-25.1593, 4.8939) (-25.2051, 4.7894) (-25.2551, 4.6862) (-25.2914, 4.6415) (-25.3542, 4.5457) (-25.4384, 4.4673) (-25.4781, 4.4265) (-25.5685, 4.3556) (-25.6659, 4.2962) (-25.7156, 4.2675) (-25.8182, 4.2166) (-25.9263, 4.1785) (-25.9809, 4.1616) (-26.0914, 4.1318) (-26.2039, 4.1105) (-26.2605, 4.1017) (-26.3741, 4.0879) (-26.4884, 4.0817) (-26.5456, 4.0804) (-26.66, 4.0807) (-26.7743, 4.0849) (-26.8314, 4.0874) (-26.9456, 4.0922) (-27.06, 4.0939) (-27.1172, 4.093) (-27.2314, 4.0895) (-27.3455, 4.0824) (-27.4026, 4.0781) (-27.5164, 4.0682) (-27.6301, 4.0562) (-27.6869, 4.0497) (-27.8003, 4.0357) (-27.9134, 4.0197) (-27.9699, 4.011) (-28.0827, 3.9929) (-28.1952, 3.9728) (-28.2514, 3.9623) (-28.3635, 3.9404) (-28.4754, 3.9169) (-28.5312, 3.9047) (-28.6427, 3.8795) (-28.7538, 3.8529) (-28.8092, 3.8391) (-28.92, 3.811) (-29.0303, 3.7814) (-29.0854, 3.7662) (-29.1954, 3.7352) (-29.305, 3.7029) (-29.3597, 3.6864) (-29.4689, 3.6528) (-29.5777, 3.6179) (-29.632, 3.6001) (-29.7404, 3.5639) (-29.8484, 3.5266) (-29.9023, 3.5076) (-30.0099, 3.4692) (-30.1171, 3.4295) (-30.1706, 3.4095) (-30.2773, 3.3688) (-30.3837, 3.3271) (-30.4369, 3.306) (-30.5428, 3.2632) (-30.6482, 3.2191) (-30.7008, 3.1968) (-30.8057, 3.1515) (-30.9102, 3.1052) (-30.9624, 3.082) (-31.0145, 3.0586) (-31.0667, 3.0352) knots 0 0 0 0 0 0 0.021315 0.021315 0.021315 0.04263 0.04263 0.04263 0.063945 0.063945 0.063945 0.08526 0.08526 0.08526 0.106575 0.106575 0.106575 0.12789 0.12789 0.12789 0.149204 0.149204 0.149204 0.170519 0.170519 0.170519 0.191835 0.191835 0.191835 0.21315 0.21315 0.21315 0.234465 0.234465 0.234465 0.255779 0.255779 0.255779 0.277094 0.277094 0.277094 0.298412 0.298412 0.298412 0.319724 0.319724 0.319724 0.341052 0.341052 0.341052 0.362374 0.362374 0.362374 0.383705 0.383705 0.383705 0.405045 0.405045 0.405045 0.42637 0.42637 0.42637 0.447676 0.447676 0.447676 0.468973 0.468973 0.468973 0.490261 0.490261 0.490261 0.511544 0.511544 0.511544 0.532795 0.532795 0.532795 0.554 0.554 0.554 0.575212 0.575212 0.575212 0.596458 0.596458 0.596458 0.617711 0.617711 0.617711 0.63897 0.63897 0.63897 0.660221 0.660221 0.660221 0.681474 0.681474 0.681474 0.702716 0.702716 0.702716 0.723962 0.723962 0.723962 0.745198 0.745198 0.745198 0.76643 0.76643 0.76643 0.787663 0.787663 0.787663 0.808897 0.808897 0.808897 0.830131 0.830131 0.830131 0.851365 0.851365 0.851365 0.872598 0.872598 0.872598 0.893831 0.893831 0.893831 0.915065 0.915065 0.915065 0.936299 0.936299 0.936299 0.957533 0.957533 0.957533 0.978766 0.978766 0.978766 1 1 1 1 1 1 projected
  arc A10 (-31.0667, 3.0352) -> (-31.1906, 1.2233) centre (0, 0) ccw projected
  spline S7 degree 5 poles (-31.1906, 1.2233) (-31.1419, 1.1929) (-31.0933, 1.1626) (-31.0446, 1.1323) (-30.947, 1.072) (-30.8488, 1.0127) (-30.7996, 0.9832) (-30.7008, 0.925) (-30.6012, 0.868) (-30.5513, 0.8398) (-30.4512, 0.7838) (-30.3506, 0.7287) (-30.3001, 0.7015) (-30.1989, 0.6475) (-30.0971, 0.5945) (-30.0461, 0.5683) (-29.9438, 0.5164) (-29.8409, 0.4657) (-29.7893, 0.4407) (-29.6859, 0.3911) (-29.5819, 0.3428) (-29.5297, 0.319) (-29.4251, 0.2719) (-29.3199, 0.2261) (-29.2672, 0.2036) (-29.1614, 0.1591) (-29.0551, 0.1161) (-29.0018, 0.0949) (-28.8949, 0.0532) (-28.7875, 0.0131) (-28.7336, -0.0066) (-28.6256, -0.0452) (-28.517, -0.0821) (-28.4626, -0.1002) (-28.3534, -0.1354) (-28.2436, -0.1687) (-28.1886, -0.1849) (-28.0782, -0.2162) (-27.9673, -0.2454) (-27.9117, -0.2595) (-27.8003, -0.2868) (-27.6884, -0.3119) (-27.6322, -0.3238) (-27.5197, -0.3462) (-27.4065, -0.3649) (-27.3498, -0.3733) (-27.2358, -0.3865) (-27.1216, -0.3973) (-27.0645, -0.4026) (-26.9503, -0.4145) (-26.8367, -0.4305) (-26.78, -0.44) (-26.6675, -0.4626) (-26.5566, -0.4926) (-26.5018, -0.5098) (-26.3932, -0.5475) (-26.2879, -0.5933) (-26.2358, -0.6179) (-26.1349, -0.6726) (-26.0401, -0.7381) (-25.9962, -0.7749) (-25.9064, -0.8469) (-25.8306, -0.9336) (-25.7949, -0.9783) (-25.7264, -1.0711) (-25.6771, -1.1748) (-25.6487, -1.2252) (-25.6165, -1.3356) (-25.5859, -1.4459) (-25.5819, -1.504) (-25.5726, -1.6176) (-25.5671, -1.7325) (-25.5621, -1.7893) (-25.5539, -1.9037) (-25.5466, -2.0176) (-25.5466, -2.0755) (-25.5626, -2.1884) (-25.5829, -2.3013) (-25.6058, -2.3541) (-25.6404, -2.4634) (-25.7004, -2.5616) (-25.7276, -2.6116) (-25.7954, -2.7043) (-25.8733, -2.7877) (-25.9133, -2.8288) (-25.9984, -2.9055) (-26.0922, -2.9712) (-26.1402, -3.0023) (-26.2387, -3.0608) (-26.3412, -3.1117) (-26.3933, -3.1354) (-26.499, -3.1793) (-26.6073, -3.2161) (-26.6621, -3.2328) (-26.7723, -3.2634) (-26.8835, -3.2902) (-26.9392, -3.3032) (-27.0505, -3.3294) (-27.161, -3.3586) (-27.2159, -3.3749) (-27.325, -3.4091) (-27.4329, -3.4468) (-27.4866, -3.4663) (-27.5937, -3.5065) (-27.6999, -3.5487) (-27.7528, -3.5703) (-27.8582, -3.6144) (-27.9628, -3.6603) (-28.0149, -3.6839) (-28.1186, -3.7318) (-28.2215, -3.7815) (-28.2728, -3.8068) (-28.3749, -3.8581) (-28.4762, -3.9109) (-28.5266, -3.9377) (-28.6272, -3.992) (-28.727, -4.0477) (-28.7767, -4.0759) (-28.8757, -4.1329) (-28.974, -4.1911) (-29.023, -4.2206) (-29.1205, -4.2801) (-29.2173, -4.3408) (-29.2656, -4.3714) (-29.3616, -4.4333) (-29.457, -4.4963) (-29.5045, -4.528) (-29.5991, -4.5921) (-29.693, -4.6572) (-29.7398, -4.69) (-29.833, -4.7561) (-29.9255, -4.8231) (-29.9716, -4.8569) (-30.0635, -4.9249) (-30.1547, -4.9937) (-30.2001, -5.0284) (-30.2906, -5.0982) (-30.3802, -5.1691) (-30.4248, -5.2048) (-30.5136, -5.2767) (-30.6018, -5.3494) (-30.6457, -5.3859) (-30.6896, -5.4224) (-30.7335, -5.459) knots 0 0 0 0 0 0 0.021315 0.021315 0.021315 0.04263 0.04263 0.04263 0.063945 0.063945 0.063945 0.08526 0.08526 0.08526 0.106575 0.106575 0.106575 0.12789 0.12789 0.12789 0.149204 0.149204 0.149204 0.170519 0.170519 0.170519 0.191835 0.191835 0.191835 0.21315 0.21315 0.21315 0.234465 0.234465 0.234465 0.255779 0.255779 0.255779 0.277094 0.277094 0.277094 0.298412 0.298412 0.298412 0.319724 0.319724 0.319724 0.341052 0.341052 0.341052 0.362374 0.362374 0.362374 0.383705 0.383705 0.383705 0.405045 0.405045 0.405045 0.42637 0.42637 0.42637 0.447676 0.447676 0.447676 0.468973 0.468973 0.468973 0.490261 0.490261 0.490261 0.511544 0.511544 0.511544 0.532795 0.532795 0.532795 0.554 0.554 0.554 0.575212 0.575212 0.575212 0.596458 0.596458 0.596458 0.617711 0.617711 0.617711 0.63897 0.63897 0.63897 0.660221 0.660221 0.660221 0.681474 0.681474 0.681474 0.702716 0.702716 0.702716 0.723962 0.723962 0.723962 0.745198 0.745198 0.745198 0.76643 0.76643 0.76643 0.787663 0.787663 0.787663 0.808897 0.808897 0.808897 0.830131 0.830131 0.830131 0.851365 0.851365 0.851365 0.872598 0.872598 0.872598 0.893831 0.893831 0.893831 0.915065 0.915065 0.915065 0.936299 0.936299 0.936299 0.957533 0.957533 0.957533 0.978766 0.978766 0.978766 1 1 1 1 1 1 projected
  arc A11 (-30.7335, -5.459) -> (-30.364, -7.2372) centre (0, 0) ccw projected
  spline S8 degree 5 poles (-30.364, -7.2372) (-30.309, -7.2533) (-30.2539, -7.2694) (-30.1989, -7.2854) (-30.0886, -7.3171) (-29.9781, -7.3478) (-29.9227, -7.3628) (-29.8119, -7.3922) (-29.7006, -7.4203) (-29.6449, -7.434) (-29.5334, -7.4609) (-29.4217, -7.4868) (-29.3657, -7.4994) (-29.2537, -7.5241) (-29.1415, -7.5476) (-29.0853, -7.5591) (-28.9728, -7.5814) (-28.86, -7.6025) (-28.8036, -7.6128) (-28.6906, -7.6325) (-28.5774, -7.651) (-28.5207, -7.6599) (-28.4073, -7.677) (-28.2937, -7.6927) (-28.2368, -7.7002) (-28.123, -7.7144) (-28.009, -7.7272) (-27.952, -7.7332) (-27.8378, -7.7445) (-27.7235, -7.7542) (-27.6663, -7.7586) (-27.5519, -7.7666) (-27.4373, -7.7729) (-27.3801, -7.7756) (-27.2654, -7.78) (-27.1508, -7.7825) (-27.0934, -7.7833) (-26.9787, -7.7836) (-26.864, -7.7818) (-26.8067, -7.7804) (-26.692, -7.7766) (-26.5775, -7.7705) (-26.5202, -7.7669) (-26.4058, -7.7581) (-26.2918, -7.7455) (-26.2349, -7.7383) (-26.1216, -7.7203) (-26.0087, -7.6998) (-25.9522, -7.6896) (-25.8391, -7.6702) (-25.7253, -7.655) (-25.6682, -7.6489) (-25.5537, -7.6402) (-25.4389, -7.6392) (-25.3815, -7.641) (-25.2668, -7.648) (-25.153, -7.6636) (-25.0962, -7.6733) (-24.9843, -7.6987) (-24.8754, -7.7362) (-24.8231, -7.7598) (-24.7172, -7.8049) (-24.6208, -7.868) (-24.5744, -7.9014) (-24.4834, -7.9723) (-24.408, -8.0588) (-24.3671, -8.0997) (-24.3063, -8.1973) (-24.247, -8.2953) (-24.2275, -8.3501) (-24.1879, -8.4571) (-24.1516, -8.5661) (-24.1314, -8.6195) (-24.0927, -8.7275) (-24.0549, -8.8352) (-24.0393, -8.8909) (-24.0243, -9.004) (-24.0133, -9.1182) (-24.0212, -9.1752) (-24.025, -9.2897) (-24.0562, -9.4005) (-24.0689, -9.4559) (-24.1093, -9.5635) (-24.1617, -9.6649) (-24.1892, -9.7152) (-24.2504, -9.812) (-24.323, -9.9006) (-24.3609, -9.9435) (-24.4399, -10.0264) (-24.5249, -10.1031) (-24.5686, -10.14) (-24.6585, -10.2108) (-24.753, -10.2755) (-24.8012, -10.3063) (-24.8991, -10.3654) (-24.9989, -10.4213) (-25.049, -10.4488) (-25.1491, -10.5041) (-25.2477, -10.562) (-25.2961, -10.5925) (-25.3919, -10.6549) (-25.4857, -10.7203) (-25.5322, -10.7535) (-25.6244, -10.8211) (-25.7152, -10.8905) (-25.7604, -10.9255) (-25.85, -10.9964) (-25.9384, -11.0689) (-25.9821, -11.1056) (-26.0691, -11.1798) (-26.1547, -11.2554) (-26.1973, -11.2935) (-26.2818, -11.3705) (-26.3651, -11.4487) (-26.4064, -11.4881) (-26.4886, -11.5675) (-26.5697, -11.648) (-26.6099, -11.6886) (-26.6899, -11.7702) (-26.7688, -11.8528) (-26.808, -11.8944) (-26.8859, -11.978) (-26.9627, -12.0626) (-27.0009, -12.1051) (-27.0767, -12.1906) (-27.1516, -12.2769) (-27.1887, -12.3203) (-27.2626, -12.4075) (-27.3354, -12.4956) (-27.3716, -12.5398) (-27.4436, -12.6285) (-27.5145, -12.7181) (-27.5498, -12.763) (-27.6199, -12.8533) (-27.6892, -12.9442) (-27.7236, -12.9898) (-27.7918, -13.0814) (-27.859, -13.1739) (-27.8923, -13.2203) (-27.9584, -13.3135) (-28.0237, -13.4073) (-28.0562, -13.4543) (-28.0886, -13.5013) (-28.121, -13.5484) knots 0 0 0 0 0 0 0.021315 0.021315 0.021315 0.04263 0.04263 0.04263 0.063945 0.063945 0.063945 0.08526 0.08526 0.08526 0.106575 0.106575 0.106575 0.12789 0.12789 0.12789 0.149204 0.149204 0.149204 0.170519 0.170519 0.170519 0.191835 0.191835 0.191835 0.21315 0.21315 0.21315 0.234465 0.234465 0.234465 0.255779 0.255779 0.255779 0.277094 0.277094 0.277094 0.298412 0.298412 0.298412 0.319724 0.319724 0.319724 0.341052 0.341052 0.341052 0.362374 0.362374 0.362374 0.383705 0.383705 0.383705 0.405045 0.405045 0.405045 0.42637 0.42637 0.42637 0.447676 0.447676 0.447676 0.468973 0.468973 0.468973 0.490261 0.490261 0.490261 0.511544 0.511544 0.511544 0.532795 0.532795 0.532795 0.554 0.554 0.554 0.575212 0.575212 0.575212 0.596458 0.596458 0.596458 0.617711 0.617711 0.617711 0.63897 0.63897 0.63897 0.660221 0.660221 0.660221 0.681474 0.681474 0.681474 0.702716 0.702716 0.702716 0.723962 0.723962 0.723962 0.745198 0.745198 0.745198 0.76643 0.76643 0.76643 0.787663 0.787663 0.787663 0.808897 0.808897 0.808897 0.830131 0.830131 0.830131 0.851365 0.851365 0.851365 0.872598 0.872598 0.872598 0.893831 0.893831 0.893831 0.915065 0.915065 0.915065 0.936299 0.936299 0.936299 0.957533 0.957533 0.957533 0.978766 0.978766 0.978766 1 1 1 1 1 1 projected
  arc A12 (-28.121, -13.5484) -> (-27.2855, -15.161) centre (0, 0) ccw projected
  arc A13 (-23.4229, -20.6329) -> (-22.1833, -21.9603) centre (0, 0) ccw projected
  arc A14 (-16.9876, -26.1872) -> (-15.4358, -27.1309) centre (0, 0) ccw projected
  arc A15 (-9.2925, -29.7993) -> (-7.5436, -30.2893) centre (0, 0) ccw projected
  arc A16 (-0.9081, -31.2014) -> (0.9081, -31.2014) centre (0, 0) ccw projected
  arc A17 (7.5436, -30.2893) -> (9.2925, -29.7993) centre (0, 0) ccw projected
  arc A18 (15.4358, -27.1309) -> (16.9876, -26.1872) centre (0, 0) ccw projected
  arc A19 (22.1833, -21.9603) -> (23.4229, -20.6329) centre (0, 0) ccw projected
  arc A20 (27.2855, -15.161) -> (28.121, -13.5484) centre (0, 0) ccw projected
  spline S9 degree 5 poles (28.121, -13.5484) (28.0885, -13.5011) (28.056, -13.4539) (28.0233, -13.4067) (27.9578, -13.3126) (27.8914, -13.219) (27.858, -13.1724) (27.7905, -13.0797) (27.722, -12.9877) (27.6874, -12.9419) (27.6179, -12.8507) (27.5475, -12.7601) (27.5121, -12.715) (27.4408, -12.6251) (27.3686, -12.536) (27.3322, -12.4917) (27.2591, -12.4033) (27.1849, -12.3158) (27.1476, -12.2723) (27.0724, -12.1856) (26.9962, -12.0999) (26.9579, -12.0572) (26.8807, -11.9724) (26.8025, -11.8885) (26.7631, -11.8468) (26.6838, -11.7639) (26.6034, -11.6821) (26.563, -11.6414) (26.4816, -11.5606) (26.399, -11.481) (26.3574, -11.4414) (26.2737, -11.363) (26.1888, -11.2859) (26.1461, -11.2476) (26.06, -11.1718) (25.9726, -11.0976) (25.9286, -11.0608) (25.8398, -10.9881) (25.7497, -10.9172) (25.7043, -10.882) (25.613, -10.8126) (25.5203, -10.745) (25.4736, -10.7118) (25.3793, -10.6464) (25.283, -10.5842) (25.2343, -10.5538) (25.135, -10.4963) (25.0345, -10.4409) (24.9842, -10.4132) (24.8843, -10.3568) (24.7864, -10.2968) (24.7382, -10.2656) (24.644, -10.2001) (24.5542, -10.1283) (24.5109, -10.0908) (24.4262, -10.0129) (24.3479, -9.929) (24.31, -9.8857) (24.2392, -9.7953) (24.1783, -9.6974) (24.1527, -9.6462) (24.099, -9.5444) (24.0641, -9.4346) (24.0491, -9.3794) (24.0233, -9.267) (24.0193, -9.1523) (24.0134, -9.0947) (24.0279, -8.9806) (24.0438, -8.8673) (24.0632, -8.8124) (24.1, -8.7044) (24.1407, -8.5969) (24.1587, -8.5428) (24.1968, -8.4346) (24.2354, -8.3272) (24.2586, -8.2741) (24.3182, -8.1769) (24.3818, -8.0814) (24.4239, -8.0421) (24.4991, -7.9557) (24.5932, -7.8895) (24.6381, -7.8545) (24.7372, -7.7966) (24.8419, -7.751) (24.895, -7.7293) (25.0036, -7.6929) (25.1158, -7.6699) (25.1723, -7.6606) (25.2858, -7.6461) (25.4001, -7.6403) (25.4574, -7.6393) (25.5718, -7.6411) (25.6859, -7.6505) (25.7427, -7.657) (25.856, -7.6729) (25.9687, -7.6926) (26.0249, -7.7029) (26.1374, -7.7232) (26.2505, -7.7405) (26.3073, -7.7473) (26.4209, -7.7594) (26.535, -7.7679) (26.592, -7.7714) (26.7062, -7.7772) (26.8204, -7.7807) (26.8776, -7.782) (26.9918, -7.7836) (27.1061, -7.7831) (27.1632, -7.7823) (27.2775, -7.7796) (27.3916, -7.775) (27.4487, -7.7723) (27.5628, -7.7659) (27.6768, -7.7578) (27.7338, -7.7533) (27.8476, -7.7436) (27.9613, -7.7323) (28.0181, -7.7262) (28.1317, -7.7134) (28.2451, -7.6991) (28.3017, -7.6916) (28.4149, -7.6759) (28.5279, -7.6588) (28.5843, -7.6499) (28.6971, -7.6314) (28.8096, -7.6117) (28.8658, -7.6015) (28.9781, -7.5804) (29.0902, -7.5581) (29.1462, -7.5467) (29.258, -7.5232) (29.3696, -7.4985) (29.4253, -7.4859) (29.5366, -7.4601) (29.6477, -7.4333) (29.7032, -7.4197) (29.814, -7.3917) (29.9244, -7.3624) (29.9796, -7.3474) (30.0897, -7.3168) (30.1995, -7.2853) (30.2543, -7.2693) (30.3092, -7.2532) (30.364, -7.2372) knots 0 0 0 0 0 0 0.021315 0.021315 0.021315 0.04263 0.04263 0.04263 0.063945 0.063945 0.063945 0.08526 0.08526 0.08526 0.106575 0.106575 0.106575 0.12789 0.12789 0.12789 0.149204 0.149204 0.149204 0.170519 0.170519 0.170519 0.191835 0.191835 0.191835 0.21315 0.21315 0.21315 0.234465 0.234465 0.234465 0.255779 0.255779 0.255779 0.277094 0.277094 0.277094 0.298412 0.298412 0.298412 0.319724 0.319724 0.319724 0.341052 0.341052 0.341052 0.362374 0.362374 0.362374 0.383705 0.383705 0.383705 0.405045 0.405045 0.405045 0.42637 0.42637 0.42637 0.447676 0.447676 0.447676 0.468973 0.468973 0.468973 0.490261 0.490261 0.490261 0.511544 0.511544 0.511544 0.532795 0.532795 0.532795 0.554 0.554 0.554 0.575212 0.575212 0.575212 0.596458 0.596458 0.596458 0.617711 0.617711 0.617711 0.63897 0.63897 0.63897 0.660221 0.660221 0.660221 0.681474 0.681474 0.681474 0.702716 0.702716 0.702716 0.723962 0.723962 0.723962 0.745198 0.745198 0.745198 0.76643 0.76643 0.76643 0.787663 0.787663 0.787663 0.808897 0.808897 0.808897 0.830131 0.830131 0.830131 0.851365 0.851365 0.851365 0.872598 0.872598 0.872598 0.893831 0.893831 0.893831 0.915065 0.915065 0.915065 0.936299 0.936299 0.936299 0.957533 0.957533 0.957533 0.978766 0.978766 0.978766 1 1 1 1 1 1 projected
  arc A21 (30.364, -7.2372) -> (30.7335, -5.459) centre (0, 0) ccw projected